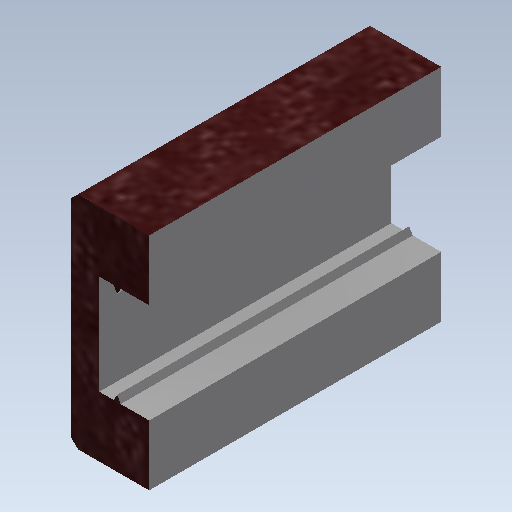
# Autodesk Inventor part: Pen_Holder
Saved by Autodesk Inventor 2021.3 (Build 253353000, 353)
## iProperties
Created: 2021-06-01
Part Number: Pen_Holder
Material: Steel, Wrought
Document SubType Name: Modeling
Designer: vivek
Density: 7.85 g/cm^3
Appearance: Steel
Author: vivek
Autodesk Inventor part; units mm, degrees
ref_plane "YZ Plane" through (0, 0, 0) normal (1, 0, 0) x (0, 1, 0)
ref_plane "XZ Plane" through (0, 0, 0) normal (0, 1, 0) x (-1, 0, 0)
ref_plane "XY Plane" through (0, 0, 0) normal (0, 0, 1) x (1, 0, 0)
sketch "Sketch1" plane through (0, 0, 0) normal (0, 0, 1) x (1, 0, 0)
  line L0 (-5.5, -15.5) -> (5.5, -15.5)
  line L1 (5.5, -15.5) -> (5.5, 15.5)
  line L2 (5.5, 15.5) -> (-5.5, 15.5)
  line L3 (-5.5, 15.5) -> (-5.5, -15.5)
  line L4 (0, 0) -> (3.6847, 0)
  line L5 (0, 0) -> (0, -8.9349)
  point P0 (5.5, 0)
  point P1 (0, -15.5)
  dimension "d0" = 11
  dimension "d1" = 31
  constraints: 12 end point, 3 perpendicular, 2 midpoint, 2 parallel, 2 point on line, 1 horizontal
  measures "d0" distance of L2.end L1.end
  measures "d1" distance of L1.end L0.end
extrude "Extrusion1" add sketch "Sketch1" along normal blind 41
sketch "Sketch2" plane through (0, 0, 41) normal (0, 0, 1) x (1, 0, 0)
  line L0 (5.5, -15.5) -> (5.5, 15.5) projected
  line L1 (5.5, -7) -> (-1.5, -7)
  line L2 (-1.5, -7) -> (-1.5, 7)
  line L3 (-1.5, 7) -> (5.5, 7)
  line L4 (5.5, 7) -> (5.5, -7)
  point P0 (0, 0)
  point P1 (5.5, 0)
  dimension "d4" = 7
  dimension "d5" = 14
  constraints: 8 end point, 2 midpoint, 2 parallel, 1 horizontal, 1 perpendicular
  measures "d4" distance of L2.end L3.end
  measures "d5" distance of L1.end L2.end
extrude "Extrusion2" cut sketch "Sketch2" against normal through all
sketch "Sketch3" plane through (0, 0, 41) normal (0, 0, 1) x (1, 0, 0)
  line L0 (-1.5, 7) -> (5.5, 7) projected
  line L1 (5.5, -7) -> (-1.5, -7) projected
  line L2 (1, 6.134) -> (0.5, 7) projected
  line L3 (0.5, 7) -> (-1.5, 7) projected
  line L4 (-1.5, -7) -> (-1.5, 7) projected
  line L5 (0.5, -7) -> (-1.5, -7) projected
  line L6 (0.5, -7) -> (1, -6.134) projected
  line L7 (1, -6.134) -> (1.5, -7) projected
  line L8 (7.5, -7) -> (1.5, -7) projected
  line L9 (7.5, 7) -> (7.5, -7) projected
  line L10 (7.5, 7) -> (1.5, 7) projected
  line L11 (1.5, 7) -> (1, 6.134) projected
  line L12 (0.5, 7) -> (1.5, 7)
  line L13 (1.5, 7) -> (1, 6.134)
  line L14 (1, 6.134) -> (0.5, 7)
  line L15 (1, -6.134) -> (1.5, -7)
  line L16 (1.5, -7) -> (0.5, -7)
  line L17 (0.5, -7) -> (1, -6.134)
  point P0 (0, 0)
  point P1 (1, 6.7113)
  point P2 (1, -6.7113)
  dimension "d8" = 1
  dimension "d9" = 1
  dimension "d10" = 2
  dimension "d11" = 2
  constraints: 12 end point, 2 collinear, 14 other
  measures "d8" distance of L15.start L15.end
  measures "d9" distance of L12.start L12.end
  measures "d10" distance from line of L4 L12.start
  measures "d11" distance of L1.end L16.end
extrude "Extrusion3" add sketch "Sketch3" against normal up to surface (41 mm away) contours L0 L11 L2 | L6 L7 L1
sketch "Sketch4" plane through (-5.5, -15.5, 0) normal (-1, 0, 0) x (0, 0, 1)
  line L0 (0, 0) -> (41, 0) projected
  line L1 (41, 31) -> (41, 0) projected
  line L2 (0, 31) -> (41, 31) projected
  circle A0 centre (30, 3) radius 1.5
  line L3 (41, 15.5) -> (23.6881, 15.5)
  line L4 (20.5, 31) -> (20.5, 20.567)
  circle A1 centre (30, 28) radius 1.5
  circle A2 centre (11, 3) radius 1.5
  circle A3 centre (11, 28) radius 1.5
  point P0 (0, 15.5)
  dimension "d14" = 3
  dimension "d15" = 3
  dimension "d16" = 11
  constraints: 4 centre point, 4 end point, 3 symmetric about line, 2 midpoint, 1 parallel, 1 perpendicular, 3 other
  measures "d14" diameter of A0
  measures "d15" distance from line of L0 A0.centre
  measures "d16" distance from line of L1 A0.centre
extrude "Extrusion4" cut sketch "Sketch4" against normal blind 3
chamfer "Chamfer1" distance 1 angle 45 2 edges at (-5.5, -15.5, 20.5) (-5.5, 15.5, 20.5)
body "Solid1"
